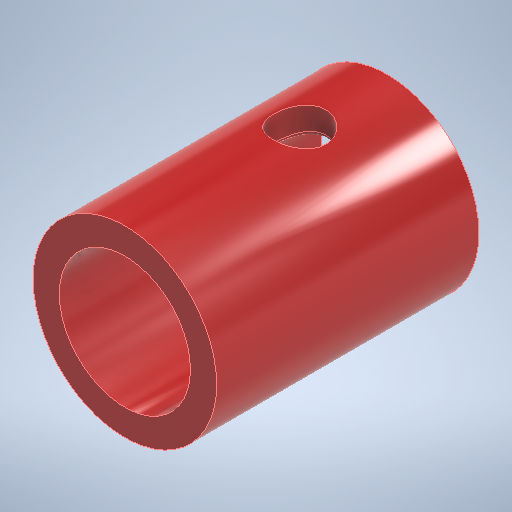
# Autodesk Inventor part: Shifter Joint
Saved by Autodesk Inventor 2025.2 (Build 292293000, 293)
## iProperties
Created: 2025-02-09
Part Number: Shifter Joint
Material: Generic
Document SubType Name: Modeling
Designer: eason
Density: 1 g/cm^3
Appearance: Red
Author: eason
Autodesk Inventor part; units mm, degrees
ref_plane "YZ Plane" through (0, 0, 0) normal (1, 0, 0) x (0, 1, 0)
ref_plane "XY Plane" through (0, 0, 0) normal (0, 0, 1) x (1, 0, 0)
sketch "Sketch1" plane through (0, 0, 0) normal (0, 0, 1) x (1, 0, 0)
  circle A0 centre (0, 0) radius 7.5
  circle A1 centre (0, 0) radius 10.5
  dimension "d0" = 15
  dimension "d1" = 3
  constraints: 2 centre point, 2 coincident
  measures "d0" diameter of A0
  measures "d1" radial gap between concentric circles of A0 A1
extrude "Extrusion1" add sketch "Sketch1" along normal blind 20 and the other way blind 10
ref_plane "Work Plane1" through (0, -10.5, 0) normal (0, 1, 0) x (-1, 0, 0)
sketch "Sketch2" plane through (0, -10.5, 0) normal (0, 1, 0) x (-1, 0, 0)
  circle A0 centre (0, 0) radius 3
  dimension "d6" = 6
  constraints: 1 centre point, 1 coincident
  measures "d6" diameter of A0
extrude "Extrusion2" cut sketch "Sketch2" along normal through all
fillet "Fillet2" radius 0.5 4 edges at (0.0002, -7.5, -3) (-0.0002, -7.5, 3) (-0.0002, 7.5, 3) (0.0002, 7.5, -3)
body "Solid1"
